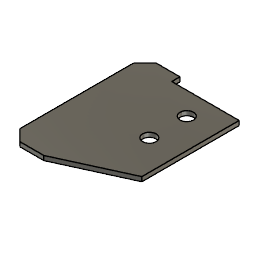
GPL H200 to H150G1 (Autodesk Fusion 360 design; units mm, degrees)
Autodesk Fusion 360 part; units mm, degrees
sketch "スケッチ1" plane through (0, 0, 0) normal (0, 0, 1) x (1, 0, 0) in component "GPL H200 to H150G1"
  line L0 (-21.5, 91) -> (-68.5, 91)
  line L1 (-68.5, 91) -> (-68.5, -91)
  line L2 (-68.5, -91) -> (-21.5, -91)
  line L3 (68.5, -50) -> (68.5, 80)
  line L4 (60.2198, 80) -> (-68.5, -91) construction
  line L5 (-68.5, 91) -> (45.5182, -60.4695) construction
  line L6 (-21.5, 91) -> (-21.5, 80)
  line L7 (-21.5, 80) -> (68.5, 80)
  line L8 (-68.5, -91) -> (-21.5, -91) construction
  line L9 (68.5, -50) -> (-21.5, -91)
  dimension "d14_1" = 18
  dimension "d15_1" = 180
  constraint horizontal L0
  constraint perpendicular L0 L1
  constraint parallel L0 L2
  constraint parallel L1 L3
  constraint coincident L4 origin
  constraint coincident L5 origin
  constraint vertical L6
  constraint horizontal L7
  constraint coincident L7 L4.start
  constraint perpendicular L3 L8
  constraint coincident L9 L5.end
  measures "d2" distance of L0.end L1.end
  measures "d5" distance of L1.end L2.end
extrude "押し出し1" add sketch "スケッチ1" along normal blind 6 makes body 1 in component "GPL H200 to H150G1"
chamfer "面取り1" distance 15 angle 45 2 edges at (-68.5, -91, 3) (-68.5, 91, 3) on bodies 1 in component "GPL H200 to H150G1"
sketch "スケッチ2" plane through (0, 0, 6) normal (0, 0, 1) x (-1, 0, 0) in component "GPL H200 to H150G1"
  line L0 (53.5, -91) -> (68.5, -76)
  line L1 (68.5, -76) -> (68.5, 76)
  line L2 (68.5, 76) -> (53.5, 91)
  line L3 (53.5, 91) -> (21.5, 91)
  line L4 (21.5, 91) -> (-68.5, 50)
  line L5 (-68.5, 50) -> (-68.5, -80)
  line L6 (-68.5, -80) -> (21.5, -80)
  line L7 (21.5, -80) -> (21.5, -91)
  line L8 (21.5, -91) -> (53.5, -91)
  line L9 (-68.5, -80) -> (-28.5, -80) construction
  line L10 (-28.5, -80) -> (-28.5, -50) construction
  line L11 (-28.5, -50) -> (-68.5, -50) construction
  line L12 (-68.5, -50) -> (-68.5, -80) construction
  line L13 (-68.5, -50) -> (-28.5, -50) construction
  line L14 (-28.5, -50) -> (-28.5, 0) construction
  line L15 (-28.5, 0) -> (-68.5, 0) construction
  line L16 (-68.5, 0) -> (-68.5, -50) construction
  point P0 (-28.5, -50)
  point P1 (-28.5, 0)
  dimension "d10" = 40
  dimension "d11" = 30
  dimension "d12" = 40
  dimension "d13" = 50
  constraint horizontal L9
  constraint vertical L10
  constraint horizontal L11
  constraint vertical L12
  constraint coincident L5.end L6.start
  constraint horizontal L13
  constraint vertical L14
  constraint horizontal L15
  constraint vertical L16
  constraint coincident P0 L10.end
  constraint coincident P1 L14.end
  measures "d10" distance of L5.end L9.end
  measures "d11" distance of L5.end L11.end
  measures "d12" distance of L11.end P0
  measures "d13" distance of L11.end L15.end
hole "穴1" at (28.5, 50, 6) at (28.5, 0, 6) direction (0, 0, -1) diameter 18 end through all bodies 1 in component "GPL H200 to H150G1"
sketch "スケッチ1 (2)" plane through (0, 0, 0) normal (0, 0, 1) x (1, 0, 0) in component "GPL　H形鋼　取付150G1 (1)"
  line L0 (-21.5, 91) -> (-68.5, 91)
  line L1 (-68.5, 91) -> (-68.5, -91)
  line L2 (-68.5, -91) -> (-21.5, -91)
  line L3 (68.5, -50) -> (68.5, 80)
  line L4 (60.2198, 80) -> (-68.5, -91) construction
  line L5 (-68.5, 91) -> (45.5182, -60.4695) construction
  line L6 (-21.5, 91) -> (-21.5, 80)
  line L7 (-21.5, 80) -> (68.5, 80)
  line L8 (-68.5, -91) -> (-21.5, -91) construction
  line L9 (68.5, -50) -> (-21.5, -91)
  dimension "d2_1" = 182
  dimension "d5_1" = 47
  constraint horizontal L0
  constraint perpendicular L0 L1
  constraint parallel L0 L2
  constraint parallel L1 L3
  constraint coincident L4 origin
  constraint coincident L5 origin
  constraint vertical L6
  constraint horizontal L7
  constraint coincident L7 L4.start
  constraint perpendicular L3 L8
  constraint coincident L9 L5.end
  measures "d2_1" distance of L0.end L1.end
  measures "d5_1" distance of L1.end L2.end
extrude "押し出し1'" add sketch "スケッチ1 (2)" along normal blind 6 separate body makes body 2 in component "GPL　H形鋼　取付150G1 (1)"
chamfer "面取り1'" distance 15 angle 45 2 edges at (-68.5, -91, 3) (-68.5, 91, 3) on bodies 2 in component "GPL　H形鋼　取付150G1 (1)"
sketch "スケッチ2 (2)" plane through (0, 0, 6) normal (0, 0, 1) x (-1, 0, 0) in component "GPL　H形鋼　取付150G1 (1)"
  line L0 (53.5, -91) -> (68.5, -76)
  line L1 (68.5, -76) -> (68.5, 76)
  line L2 (68.5, 76) -> (53.5, 91)
  line L3 (53.5, 91) -> (21.5, 91)
  line L4 (21.5, 91) -> (-68.5, 50)
  line L5 (-68.5, 50) -> (-68.5, -80)
  line L6 (-68.5, -80) -> (21.5, -80)
  line L7 (21.5, -80) -> (21.5, -91)
  line L8 (21.5, -91) -> (53.5, -91)
  line L9 (-68.5, -80) -> (-28.5, -80) construction
  line L10 (-28.5, -80) -> (-28.5, -50) construction
  line L11 (-28.5, -50) -> (-68.5, -50) construction
  line L12 (-68.5, -50) -> (-68.5, -80) construction
  line L13 (-68.5, -50) -> (-28.5, -50) construction
  line L14 (-28.5, -50) -> (-28.5, 0) construction
  line L15 (-28.5, 0) -> (-68.5, 0) construction
  line L16 (-68.5, 0) -> (-68.5, -50) construction
  point P0 (-28.5, -50)
  point P1 (-28.5, 0)
  dimension "d10_1" = 40
  dimension "d11_1" = 30
  dimension "d12_1" = 40
  dimension "d13_1" = 50
  constraint horizontal L9
  constraint vertical L10
  constraint horizontal L11
  constraint vertical L12
  constraint coincident L5.end L6.start
  constraint horizontal L13
  constraint vertical L14
  constraint horizontal L15
  constraint vertical L16
  constraint coincident P0 L10.end
  constraint coincident P1 L14.end
  measures "d10_1" distance of L5.end L9.end
  measures "d11_1" distance of L5.end L11.end
  measures "d12_1" distance of L11.end P0
  measures "d13_1" distance of L11.end L15.end
hole "穴1'" at (28.5, 50, 6) at (28.5, 0, 6) direction (0, 0, -1) diameter 18 end through all bodies 2 in component "GPL　H形鋼　取付150G1 (1)"
component "GPL H200 to H150G1" placed x (1, 0, 0) y (0, 1, 0) z (0, 0, 1) at (0, 0, 0)
equation "d5 = 15 mm + 32 mm"
equation "d5_1 = 15 mm + 32 mm"
